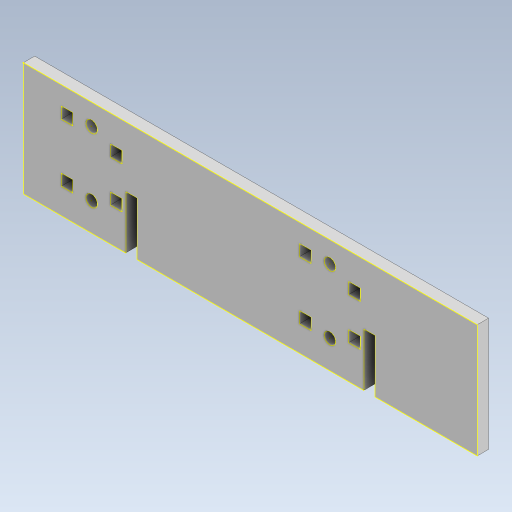
# Autodesk Inventor part: 零件8
Saved by Autodesk Inventor 2023 (Build 270158000, 158)
## iProperties
Created: 2023-05-16
Part Number: 零件8
Material: 一般
Document SubType Name: Modeling
Designer: Johnny Jou
Density: 1 g/cm^3
Appearance: 預設
Author: Johnny Jou
Autodesk Inventor part; units mm, degrees
ref_plane "YZ Plane" through (0, 0, 0) normal (1, 0, 0) x (0, 1, 0)
ref_plane "XZ Plane" through (0, 0, 0) normal (0, 1, 0) x (-1, 0, 0)
ref_plane "XY Plane" through (0, 0, 0) normal (0, 0, 1) x (1, 0, 0)
sketch "草圖1" plane through (0, 0, 0) normal (0, 0, 1) x (1, 0, 0)
  line L0 (0, 0) -> (120, 0)
  line L1 (120, 0) -> (120, -27)
  line L2 (120, -27) -> (0, -27)
  line L3 (0, -27) -> (0, 0)
  line L4 (27.05, -27) -> (30, -27)
  line L5 (30, -27) -> (30, -16)
  line L6 (30, -16) -> (27.05, -16)
  line L7 (27.05, -16) -> (27.05, -27)
  line L8 (90, -27) -> (92.95, -27)
  line L9 (92.95, -27) -> (92.95, -16)
  line L10 (92.95, -16) -> (90, -16)
  line L11 (90, -16) -> (90, -27)
  line L12 (30, -16) -> (90, -16)
  point P0 (60, -16)
  point P1 (60, -27)
  dimension "d0" = 60
  dimension "d1" = 120
  dimension "d2" = 2.95
  dimension "d3" = 2.95
  dimension "d4" = 11
  dimension "d5" = 27
  constraints: 26 end point, 6 parallel, 4 perpendicular, 4 point on line, 2 midpoint, 1 horizontal, 1 vertical alignment
  measures "d0" distance between parallel lines of L11 L5
  measures "d1" distance of L1.end L2.end
  measures "d2" distance of L9.end L10.end
  measures "d3" distance of L5.end L6.end
  measures "d4" distance of L6.end L4.start
  measures "d5" distance of L0.end L1.end
extrude "擠出1" add sketch "草圖1" along normal blind 3 contours L0 L1 L2 L9 L10 L12 L6 L7 L3 | L5 L12 L11 L2
sketch "草圖2" plane through (0, 0, 3) normal (0, 0, 1) x (1, 0, 0)
  line L0 (13, -23.2937) -> (13, -20.2937)
  line L1 (13, -20.2937) -> (10, -20.2937)
  line L2 (10, -23.2937) -> (10, -20.2937)
  line L3 (13, -23.2937) -> (10, -23.2937)
  line L4 (26, -18.1103) -> (26, -21.1103)
  line L5 (23, -18.1103) -> (23, -21.1103)
  line L6 (23, -21.1103) -> (26, -21.1103)
  line L7 (23, -18.1103) -> (26, -18.1103)
  line L8 (26, -7.1103) -> (26, -10.1103)
  line L9 (23, -10.1103) -> (26, -10.1103)
  line L10 (23, -7.1103) -> (23, -10.1103)
  line L11 (23, -7.1103) -> (26, -7.1103)
  line L12 (10, -7.9269) -> (13, -7.9269)
  line L13 (13, -4.9269) -> (13, -7.9269)
  line L14 (10, -4.9269) -> (13, -4.9269)
  line L15 (10, -4.9269) -> (10, -7.9269)
  line L16 (24.5, -18.1103) -> (24.5, -10.1103) construction
  line L17 (0, 0) -> (0, -27) projected
  line L18 (11.5, -20.2937) -> (11.5, -7.9269) construction
  line L19 (27.05, -27) -> (27.05, -16) projected
  line L20 (26, -19.6103) -> (27.05, -19.6103) construction
  circle A0 centre (18, -22.6103) radius 1.5
  circle A1 centre (18, -5.6103) radius 1.5
  point P0 (11.5, -4.9269)
  point P1 (24.5, -14.1103)
  point P2 (0, -13.5)
  point P3 (11.5, -14.1103)
  point P4 (0, -13.5)
  point P5 (0, -13.5)
  dimension "d8" = 3
  dimension "d9" = 3
  dimension "d10" = 10
  dimension "d11" = 8
  dimension "d12" = 2.1834
  dimension "d13" = 2.1834
  dimension "d17" = 1.05
  dimension "d18" = 0.6103
  dimension "d27" = 3
  dimension "d28" = 5
  dimension "d29" = 0.6834
  dimension "d30" = 5
  dimension "d31" = 0.6834
  constraints: 38 end point, 11 midpoint, 9 equal length, 9 perpendicular, 2 centre point, 2 collinear, 1 equal radius, 1 horizontal alignment, 1 point on line
  measures "d8" distance of L0.start L2.start
  measures "d9" distance of L2.start L1.end
  measures "d10" distance between parallel lines of L5 L0
  measures "d11" distance between parallel lines of L9 L7
  measures "d12" distance between parallel lines of L3 L6
  measures "d13" distance from line of point (11.5, -4.927) L11
  measures "d17" distance of L20.start L20.end
  measures "d18" vertical distance of point (0, -13.5) point (11.5, -14.11)
  measures "d27" diameter of A0
  measures "d28" distance from line of L0 A0.centre
  measures "d29" distance from line of L3 A0.centre
  measures "d30" distance from line of L13 A1.centre
  measures "d31" distance from line of L14 A1.centre
extrude "擠出2" cut sketch "草圖2" against normal up to surface (3 mm away)
pattern_linear "矩形陣列1" count 2 spacing 63 along (1, 0, 0) of "擠出2"
sketch "草圖4" plane through (0, 0, 3) normal (0, 0, 1) x (1, 0, 0)
  line L0 (0, -27) -> (27.05, -27) projected
  line L1 (0, -27) -> (120, -27)
  line L2 (120, -27) -> (120, -30.0376)
  line L3 (120, -30.0376) -> (0, -30.0376)
  line L4 (0, -30.0376) -> (0, -27)
  line L5 (120, -27) -> (120, 0) projected
  line L6 (90, -27) -> (90, -16) projected
  line L7 (90, -27) -> (90, -30.0376)
  line L8 (92.95, -16) -> (92.95, -27) projected
  line L9 (92.95, -27) -> (92.95, -30.0376)
  line L10 (27.05, -27) -> (27.05, -30.0376)
  line L11 (30, -27) -> (90, -27) projected
  line L12 (30, -27) -> (30, -30.0376)
  point P0 (0, 0)
  point P1 (120, -3)
  constraints: 16 end point, 5 perpendicular, 4 point on line, 2 parallel, 1 collinear, 1 horizontal
extrude "擠出4" add sketch "草圖4" against normal up to surface (3 mm away) contours L0 L10 L3 L4 | L1 L7 L3 L12 | L1 L2 L3 L9
sketch "草圖5" plane through (0, 0, 3) normal (0, 0, 1) x (1, 0, 0)
  line L0 (89, -10.1103) -> (86, -10.1103) projected
  line L1 (86, -10.1103) -> (86, -7.1103) projected
  line L2 (86, -7.1103) -> (89, -7.1103) projected
  line L3 (89, -7.1103) -> (89, -10.1103) projected
  circle A0 centre (81, -5.6103) radius 1.5 projected
  line L4 (89, -21.1103) -> (86, -21.1103) projected
  line L5 (86, -21.1103) -> (86, -18.1103) projected
  line L6 (86, -18.1103) -> (89, -18.1103) projected
  line L7 (89, -18.1103) -> (89, -21.1103) projected
  line L8 (76, -23.2937) -> (73, -23.2937) projected
  line L9 (73, -23.2937) -> (73, -20.2937) projected
  line L10 (73, -20.2937) -> (76, -20.2937) projected
  line L11 (76, -20.2937) -> (76, -23.2937) projected
  circle A1 centre (81, -22.6103) radius 1.5 projected
  line L12 (76, -7.9269) -> (73, -7.9269) projected
  line L13 (73, -7.9269) -> (73, -4.9269) projected
  line L14 (73, -4.9269) -> (76, -4.9269) projected
  line L15 (76, -4.9269) -> (76, -7.9269) projected
  line L16 (26, -10.1103) -> (23, -10.1103) projected
  line L17 (23, -10.1103) -> (23, -7.1103) projected
  line L18 (23, -7.1103) -> (26, -7.1103) projected
  line L19 (26, -7.1103) -> (26, -10.1103) projected
  circle A2 centre (18, -5.6103) radius 1.5 projected
  line L20 (26, -21.1103) -> (23, -21.1103) projected
  line L21 (23, -21.1103) -> (23, -18.1103) projected
  line L22 (23, -18.1103) -> (26, -18.1103) projected
  line L23 (26, -18.1103) -> (26, -21.1103) projected
  line L24 (13, -23.2937) -> (10, -23.2937) projected
  line L25 (10, -23.2937) -> (10, -20.2937) projected
  line L26 (10, -20.2937) -> (13, -20.2937) projected
  line L27 (13, -20.2937) -> (13, -23.2937) projected
  circle A3 centre (18, -22.6103) radius 1.5 projected
  line L28 (13, -7.9269) -> (10, -7.9269) projected
  line L29 (10, -7.9269) -> (10, -4.9269) projected
  line L30 (10, -4.9269) -> (13, -4.9269) projected
  line L31 (13, -4.9269) -> (13, -7.9269) projected
  line L32 (120, 0) -> (0, 0) projected
  line L33 (0, 0) -> (0, -30.0376) projected
  line L34 (0, -30.0376) -> (27.05, -30.0376) projected
  line L35 (27.05, -30.0376) -> (27.05, -16) projected
  line L36 (27.05, -16) -> (30, -16) projected
  line L37 (30, -16) -> (30, -30.0376) projected
  line L38 (30, -30.0376) -> (90, -30.0376) projected
  line L39 (90, -30.0376) -> (90, -16) projected
  line L40 (90, -16) -> (92.95, -16) projected
  line L41 (92.95, -16) -> (92.95, -30.0376) projected
  line L42 (92.95, -30.0376) -> (120, -30.0376) projected
  line L43 (120, -30.0376) -> (120, 0) projected
equation "\"d13\" = d12"
equation "\"d30\" = d28"
equation "\"d31\" = d29"
